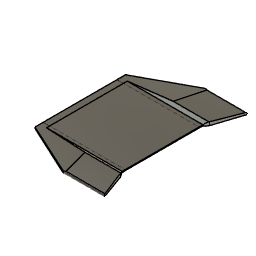
Downey-X-43A_wings v4 (Autodesk Fusion 360 design; units mm, degrees)
Autodesk Fusion 360 part; units mm, degrees
note: some values were not read from the file. Set by a fixed rule: which sketch regions a step uses.
sketch "Sketch9" plane through (0, 0, 0) normal (0, 0, 1) x (1, 0, 0)
  line L0 (3776.472, 1266.444) -> (3776.472, -304.8)
  line L1 (3776.472, 480.822) -> (2072.6401, 480.822)
  line L2 (3775.8634, 1264.9224) -> (3651.504, 954.024)
  line L3 (3651.504, 954.024) -> (3624.7105, 915.963)
  line L4 (2627.376, 883.92) -> (2761.488, 963.168)
  line L5 (2761.488, 963.168) -> (3394.4421, 1266.444)
  line L6 (3394.4421, 1266.444) -> (3775.8634, 1264.9224)
  line L7 (3775.8634, -303.2784) -> (3651.504, 7.62)
  line L8 (3651.504, 7.62) -> (3624.7105, 45.681)
  line L9 (2761.488, -1.524) -> (3394.4421, -304.8)
  line L10 (3394.4421, -304.8) -> (3775.8634, -303.2784)
  line L11 (2627.376, 77.724) -> (2761.488, -1.524)
  line L12 (2627.376, 883.92) -> (2627.376, 77.724)
  line L13 (3624.7105, 915.963) -> (3624.7105, 45.681)
  point P0 (3776.472, -304.8)
  constraint vertical L0
  constraint midpoint L0 L1.start
  constraint perpendicular L0 L1
  constraint symmetric L0.start L1 P0
  constraint symmetric L1 L2.end L7.end
  constraint symmetric L1 L3.end L8.end
  constraint symmetric L1 L4.start L11.start
  constraint symmetric L1 L4.end L9.start
  constraint symmetric L1 L5.end L9.end
  constraint symmetric L1 L2.start L7.start
extrude "Extrude6" add sketch "Sketch9" along normal blind 213.36
sketch "Sketch10" plane through (0, 0, 0) normal (1, 0, 0) x (0, 1, 0)
  line L0 (1266.444, 220.98) -> (-304.8, 220.98) construction
  line L1 (480.822, 220.98) -> (480.822, -213.36)
  line L2 (908.185, 131.0434) -> (947.928, 149.352)
  line L3 (947.928, 149.352) -> (1225.8609, 152.5533)
  line L4 (1228.3549, 130.0128) -> (926.592, 112.776)
  line L5 (926.592, 112.776) -> (908.304, 118.872)
  arc A0 (1226.8338, 129.9259) -> (1225.8609, 152.5533) centre (1226.9491, 141.2655) ccw
  line L6 (908.185, 131.0434) -> (871.728, 131.0434)
  line L7 (871.728, 231.648) -> (1286.256, 231.648)
  line L8 (1286.256, 231.648) -> (1286.256, -12.192)
  line L9 (1286.256, -12.192) -> (871.728, -12.192)
  line L10 (871.728, 121.92) -> (908.304, 118.872)
  line L11 (53.459, 131.0434) -> (89.916, 131.0434)
  line L12 (53.459, 131.0434) -> (13.716, 149.352)
  line L13 (13.716, 149.352) -> (-264.2169, 152.5533)
  arc A1 (-264.2169, 152.5533) -> (-265.1898, 129.9259) centre (-265.3051, 141.2655) ccw
  line L14 (-266.7108, 130.0128) -> (35.052, 112.776)
  line L15 (35.052, 112.776) -> (53.34, 118.872)
  line L16 (89.916, 121.92) -> (53.34, 118.872)
  line L17 (-324.612, -12.192) -> (89.916, -12.192)
  line L18 (-324.612, 231.648) -> (-324.612, -12.192)
  line L19 (89.916, 231.648) -> (-324.612, 231.648)
  line L20 (871.728, 231.648) -> (89.916, 231.648)
  line L21 (871.728, -12.192) -> (89.916, -12.192)
  line L22 (871.728, 121.92) -> (89.916, 121.92)
  line L23 (871.728, 131.0434) -> (89.916, 131.0434)
  constraint horizontal L0
  constraint midpoint L0 L1.start
  constraint perpendicular L0 L1
  constraint coincident L4.start A0
  constraint coincident L4 A0.start
  constraint parallel L0 L6
  constraint perpendicular L7 L8
  constraint symmetric L1 L2.start L11.start
  constraint symmetric L1 L2.end L12.end
  constraint symmetric L1 L3.end L13.end
  constraint symmetric L1 L4.start L14.start
  constraint symmetric L1 L4.end L14.end
  constraint symmetric L1 L5.end L15.end
  constraint symmetric L1 A0.start A1.end
  constraint symmetric L1 A0 A1
  constraint symmetric L1 L6.end L11.end
  constraint symmetric L1 L7.start L19.start
  constraint symmetric L1 L7.end L18.start
  constraint symmetric L1 L8.end L17.start
  constraint symmetric L1 L9.end L17.end
  constraint symmetric L1 L10.start L16.start
  constraint parallel L9 L21
  constraint parallel L11 L23
extrude "Extrude7" cut sketch "Sketch10" along normal blind 4145.28
sketch "Sketch11" plane through (0, 0, 0) normal (0, 1, 0) x (1, 0, 0)
  line L0 (2590.8001, -213.36) -> (3810.0001, -213.36)
  line L1 (3810.0001, -213.36) -> (3810.0001, -30.48)
  line L2 (3810.0001, -30.48) -> (2590.8001, -30.48)
  line L3 (2590.8001, -30.48) -> (2590.8001, -213.36)
  line L4 (2753.8681, -128.1304) -> (2753.8681, -112.776)
  line L5 (2753.8681, -112.776) -> (3346.704, -91.44)
  line L6 (3346.704, -91.44) -> (3779.5201, -91.44)
  line L7 (3779.5201, -91.44) -> (3779.5201, -170.688)
  line L8 (2753.8681, -128.1304) -> (3493.008, -158.496)
  line L9 (3493.008, -158.496) -> (3779.5201, -170.688)
  constraint horizontal L0
  constraint vertical L1
  constraint horizontal L2
  constraint vertical L3
  constraint vertical L4
  constraint perpendicular L4 L6
  constraint perpendicular L6 L7
extrude "Extrude8" cut sketch "Sketch11" along normal mid plane 3108.96
